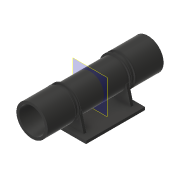
# Autodesk Inventor part: 00_Sensirion_Flowsensor
Saved by Autodesk Inventor 2019.4 (Build 234330000, 330)
## iProperties
Created: 2021-06-01
Part Number: 00_Sensirion_Flowsensor
Material: Generic
Document SubType Name: Modeling
Designer: diederichbenedict
Density: 1 g/cm^3
Appearance: Smooth - Black
Author: diederichbenedict
Autodesk Inventor part; units mm, degrees
ref_plane "YZ Plane" through (0, 0, 0) normal (1, 0, 0) x (0, 1, 0)
ref_plane "XZ Plane" through (0, 0, 0) normal (0, 1, 0) x (-1, 0, 0)
ref_plane "XY Plane" through (0, 0, 0) normal (0, 0, 1) x (1, 0, 0)
sketch "Sketch1" plane through (0, 0, 0) normal (0, 1, 0) x (-1, 0, 0)
  line L0 (0, 0) -> (0, 21.25)
  line L1 (0, 21.25) -> (0, 41.25)
  line L2 (0, 41.25) -> (11, 41.25)
  line L3 (11, 41.25) -> (11, 21.25)
  line L4 (11, 21.25) -> (9.9, 21.25)
  line L5 (9.9, 21.25) -> (9.9, 18.75)
  line L6 (9.9, 18.75) -> (11, 18.75)
  line L7 (11, 18.75) -> (11, 17.75)
  line L8 (11, 17.75) -> (9.9, 17.75)
  line L9 (9.9, 17.75) -> (9.9, 0)
  line L10 (9.9, 0) -> (0, 0)
  dimension "d1" = 20
  dimension "d2" = 11
  dimension "d3" = 20
  dimension "d4" = 9.9
  dimension "d6" = 2.5
  dimension "d7" = 1
  dimension "d8" = 0
  dimension "d19" = 17.75
  constraints: 22 end point, 6 perpendicular, 2 parallel, 2 point on line, 1 vertical
  measures "d1" distance of L0.end L1.end
  measures "d2" distance of L1.end L2.end
  measures "d3" distance of L2.end L3.end
  measures "d4" distance of L9.end L0.start
  measures "d6" distance between parallel lines of L6 L4
  measures "d7" distance between parallel lines of L8 L6
  measures "d8" distance between parallel lines of L7 L3
  measures "d19" distance from line of L9.end L8
revolve "Revolution1" add sketch "Sketch1" angle 360 about axis through (0, 0, 21.25) along (0, 0, 1)
sketch "Sketch2" plane through (0, 0, 41.25) normal (0, 0, 1) x (1, 0, 0)
  circle A0 centre (0, 0) radius 11 projected
  circle A1 centre (0, 0) radius 9.2
  point P0 (0, 0)
  dimension "d20" = 1.8
  constraints: 1 centre point, 1 coincident
  measures "d20" radial gap between concentric circles of A1 A0
extrude "Extrusion1" cut sketch "Sketch2" against normal through all draft -5 contours A1
mirror "Mirror1" about plane through (0, 0, 0) normal (0, 0, -1) of "Revolution1", "Extrusion1"
ref_plane "Work Plane1" through (0, 0, 0) normal (0, 0, -1) x (-1, 0, 0)
sketch "Sketch3" plane through (0, 0, 17.75) normal (0, 0, -1) x (-1, 0, 0)
  circle A0 centre (0, 0) radius 5.5911 projected
  circle A1 centre (0, 0) radius 9.2 projected
  circle A2 centre (0, 0) radius 9.9 projected
  line L0 (-9.855, -0.943) -> (-13.2196, -13.5)
  line L1 (-9.855, -0.943) -> (3.145, -0.943) construction
  line L2 (9.8922, -0.393) -> (13.4042, -13.5)
  line L3 (9.8922, -0.393) -> (23.4616, -0.393) construction
  line L4 (13.4042, -13.5) -> (-13.2196, -13.5)
  point P0 (0, 0)
  dimension "d12" = 13
  dimension "d13" = 105
  dimension "d14" = 75
  dimension "d21" = 13.5
  constraints: 10 end point, 3 horizontal, 2 equal length, 2 point on circle
  measures "d12" distance of L0.start L0.end
  measures "d13" angle of L0 L1
  measures "d14" angle of L2 L3
  measures "d21" distance from line of L4 point (0, 0)
extrude "Extrusion2" add sketch "Sketch3" along normal blind 2 contours A2 L2 L4 L0
mirror "Mirror2" about plane through (0, 0, 0) normal (0, 0, -1) of "Extrusion2"
sketch "Sketch4" plane through (-13.4042, -13.5, -17.75) normal (0, -1, 0) x (1, 0, 0)
  line L0 (26.6239, 0) -> (0, 0) projected
  line L1 (26.6239, 0) -> (26.6239, 2) projected
  line L2 (26.6239, 2) -> (0, 2) projected
  line L3 (0, 0) -> (0, 2) projected
  line L4 (26.6239, 35.5) -> (0, 35.5) projected
  line L5 (0, 35.5) -> (0, 33.5) projected
  line L6 (26.6239, 33.5) -> (0, 33.5) projected
  line L7 (26.6239, 35.5) -> (26.6239, 33.5) projected
  line L8 (31.4495, -3.0996) -> (-4.641, -3.0996)
  line L9 (-4.641, -3.0996) -> (-4.641, 38.5996)
  line L10 (-4.641, 38.5996) -> (31.4495, 38.5996)
  line L11 (31.4495, 38.5996) -> (31.4495, -3.0996)
  line L12 (31.4495, -3.0996) -> (-4.641, 38.5996) construction
  line L13 (-4.641, -3.0996) -> (31.4495, 38.5996) construction
  point P0 (13.4042, 17.75)
  constraints: 12 end point, 2 midpoint, 2 parallel, 1 horizontal, 1 perpendicular
extrude "Extrusion3" add sketch "Sketch4" along normal blind 2
body "Solid1"
